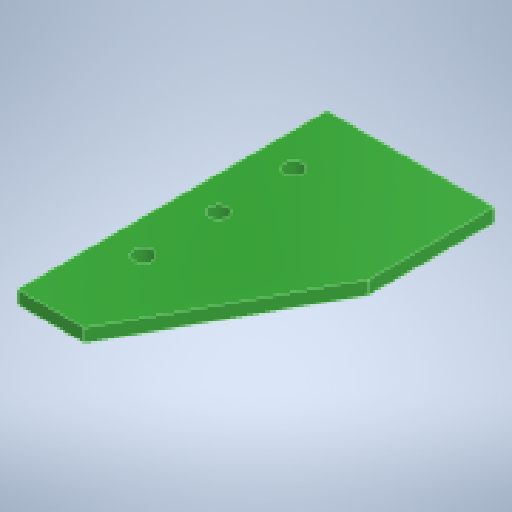
# Autodesk Inventor part: probe_PCB
Saved by Autodesk Inventor 2024.1 (Build 281209000, 209)
## iProperties
Created: 2023-10-06
Part Number: probe_PCB
Material: Generic
Document SubType Name: Modeling
Designer: l1534
Density: 1 g/cm^3
Appearance: Smooth - Dark Forest Green
Author: l1534
Autodesk Inventor part; units mm, degrees
ref_plane "YZ Plane" through (0, 0, 0) normal (1, 0, 0) x (0, 1, 0)
ref_plane "XZ Plane" through (0, 0, 0) normal (0, 1, 0) x (-1, 0, 0)
ref_plane "XY Plane" through (0, 0, 0) normal (0, 0, 1) x (1, 0, 0)
sketch "Sketch1" plane through (0, 0, 0) normal (0, 1, 0) x (-1, 0, 0)
  line L0 (18.0182, 9.2095) -> (18.0182, -27.7905)
  line L1 (18.0182, -27.7905) -> (-1.9818, -27.7905)
  line L2 (-1.9818, -27.7905) -> (-1.9818, -12.7905)
  line L3 (-1.9818, -12.7905) -> (10.0182, 9.2095)
  line L4 (10.0182, 9.2095) -> (18.0182, 9.2095)
  point P0 (0, 0)
  dimension "d0" = 37
  dimension "d1" = 8
  dimension "d2" = 20
  dimension "d3" = 15
  constraints: 10 end point, 2 perpendicular, 1 parallel, 1 vertical
  measures "d0" distance of L0.start L0.end
  measures "d1" distance of L3.end L0.start
  measures "d2" distance of L0.end L1.end
  measures "d3" distance of L1.end L2.end
extrude "Extrusion1" add sketch "Sketch1" along normal blind 1.6
sketch "Sketch2" plane through (0, 0, 0) normal (0, -1, 0) x (1, 0, 0)
  circle A0 centre (-14.0182, -10.7905) radius 1.1
  circle A1 centre (-14.0182, -19.7905) radius 1.1
  line L0 (-18.0182, -27.7905) -> (-18.0182, 9.2095) projected
  line L1 (1.9818, -27.7905) -> (-18.0182, -27.7905) projected
  circle A2 centre (-14.0182, -1.7905) radius 1.1
  point P0 (0, 0)
  dimension "d6" = 2.2
  dimension "d7" = 2.2
  dimension "d8" = 4
  dimension "d9" = 4
  dimension "d10" = 8
  dimension "d11" = 9
  dimension "d14" = 2.2
  dimension "d15" = 4
  dimension "d16" = 9
  constraints: 3 centre point
  measures "d6" diameter of A0
  measures "d7" diameter of A1
  measures "d8" distance from line of L0 A0.centre
  measures "d9" distance from line of L0 A1.centre
  measures "d10" distance from line of L1 A1.centre
  measures "d11" distance of A1.centre A0.centre
  measures "d14" diameter of A2
  measures "d15" distance from line of L0 A2.centre
  measures "d16" distance of A0.centre A2.centre
extrude "Extrusion2" cut sketch "Sketch2" against normal through all
body "Solid1"
